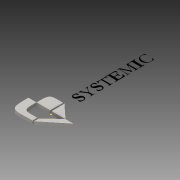
# Autodesk Inventor part: Systemic_Logo
Saved by Autodesk Inventor 2016 (Build 200138000, 138)
## iProperties
Created: 2015-05-10
Part Number: Systemic_Logo
Material: Generic
Document SubType Name: Modeling
Designer: Yann
Density: 1 g/cm^3
Appearance: Aluminum - Polished
Author: Yann
Autodesk Inventor part; units mm, degrees
ref_plane "YZ Plane" through (0, 0, 0) normal (1, 0, 0) x (0, 1, 0)
ref_plane "XZ Plane" through (0, 0, 0) normal (0, 1, 0) x (-1, 0, 0)
ref_plane "XY Plane" through (0, 0, 0) normal (0, 0, 1) x (1, 0, 0)
sketch "Sketch1" plane through (0, 0, 0) normal (0, 1, 0) x (-1, 0, 0)
  line L0 (6.9821, 0) -> (4.4821, 0)
  line L1 (0.2, 4) -> (0.2, 5.5)
  line L2 (-4.4821, 0) -> (-6.9821, 0)
  line L3 (-0.2, 5.5) -> (-0.2, 4)
  line L4 (-10.1992, 0) -> (12.3203, 0) construction
  line L5 (0, -41.6633) -> (0, 16.1649) construction
  line L6 (0.2, 5.5) -> (0.4844, 5.5) construction
  line L7 (0.4844, 5.5) -> (6.9821, 5.5) construction
  line L8 (6.9821, 5.5) -> (6.9821, 6.8061) construction
  line L9 (6.9821, 6.8061) -> (6.9821, 0) construction
  spline S0 degree 4 poles (0.2, 5.5) (0.4844, 5.5) (6.9821, 5.5) (6.9821, 6.8061) (6.9821, 0) knots 1 1 1 1 1 2 2 2 2 2
  line L10 (0.2, 4) -> (1.0687, 4) construction
  line L11 (1.0687, 4) -> (4.4821, 4) construction
  line L12 (4.4821, 4) -> (4.4821, 4.6412) construction
  line L13 (4.4821, 4.6412) -> (4.4821, 0) construction
  spline S1 degree 4 poles (0.2, 4) (1.0687, 4) (4.4821, 4) (4.4821, 4.6412) (4.4821, 0) knots 1 1 1 1 1 2 2 2 2 2
  line L14 (0.2, 4) -> (-0.2, 4) construction
  line L15 (-0.2, 5.5) -> (-6.9821, 0)
  line L16 (4.4821, 0) -> (0.2, 0)
  line L17 (-4.4821, 0) -> (-0.2, 0)
  line L18 (-0.2, 0) -> (-0.2, -4)
  line L19 (-0.2, -4) -> (-4.4821, 0)
  line L20 (0.2, -4) -> (1.0687, -4) construction
  line L21 (1.0687, -4) -> (4.4821, -4) construction
  line L22 (4.4821, -4) -> (4.4821, -4.6412) construction
  line L23 (4.4821, -4.6412) -> (4.4821, 0) construction
  spline S2 degree 4 poles (0.2, -4) (1.0687, -4) (4.4821, -4) (4.4821, -4.6412) (4.4821, 0) knots 1 1 1 1 1 2 2 2 2 2
  line L24 (0.2, 0) -> (0.2, -4)
  line L25 (-0.2, -4) -> (0.2, -4) construction
  line L26 (-4.4821, 0) -> (-0.2, 4)
  point P0 (0, 0)
  dimension "d0" = 0.2
  dimension "d1" = 4
  dimension "d3" = 2.5
  dimension "d6" = 1.5
  constraints: 26 end point, 5 perpendicular, 5 symmetric about line, 4 horizontal, 4 point on line, 4 vertical, 2 collinear, 2 equal length, 1 parallel, 11 other
  measures "d0" distance between parallel lines of L5 L1
  measures "d1" vertical distance of L1.start point (0, 0)
  measures "d3" distance of L2.start L2.end
  measures "d6" distance of L3.start L3.end
extrude "Extrusion1" add sketch "Sketch1" along normal blind 1
sketch "Sketch2" plane through (0, 0, 0) normal (0, 1, 0) x (-1, 0, 0)
  line L0 (0, -40.0826) -> (0, 6.6804) construction
  line L1 (-5.6893, 0) -> (7.9729, 0) construction
  spline S0 degree 4 poles (5.7309, -9.156) (6.4153, -8.9173) (4.9983, -7.4481) (5.0462, -8.6728) (4.0888, -9.5797) (3.7167, -8.7652) (3.7309, -8.156) knots 0 0 0 0 0 0.475399 0.676528 1 1 1 1 1
  line L2 (3.7203, -8.6135) -> (3.7416, -7.6985) construction
  arc A0 (3.7712, -7.7964) -> (3.7544, -8.5171) centre (5.7845, -8.2039) ccw construction
  point P0 (0, 0)
  point P1 (2.7309, -8.156)
  point P2 (2.7309, -9.156)
  point P3 (3.7309, -9.156)
  point P4 (4.7309, -8.156)
  point P5 (4.7309, -9.156)
  point P6 (5.7309, -8.156)
  point P7 (2.7309, -10.156)
  point P8 (3.7309, -10.156)
  point P9 (4.7309, -10.156)
  point P10 (5.7309, -10.156)
  point P11 (2.7309, -11.156)
  point P12 (3.7309, -11.156)
  point P13 (4.7309, -11.156)
  point P14 (5.7309, -11.156)
  point P15 (2.7309, -12.156)
  point P16 (3.7309, -12.156)
  point P17 (4.7309, -12.156)
  point P18 (5.7309, -12.156)
  point P19 (2.7309, -13.156)
  point P20 (3.7309, -13.156)
  point P21 (4.7309, -13.156)
  point P22 (5.7309, -13.156)
  point P23 (2.7309, -14.156)
  point P24 (3.7309, -14.156)
  point P25 (4.7309, -14.156)
  point P26 (5.7309, -14.156)
  point P27 (2.7309, -15.156)
  point P28 (3.7309, -15.156)
  point P29 (4.7309, -15.156)
  point P30 (5.7309, -15.156)
  point P31 (2.7309, -16.156)
  point P32 (3.7309, -16.156)
  point P33 (4.7309, -16.156)
  point P34 (5.7309, -16.156)
  point P35 (2.7309, -17.156)
  point P36 (3.7309, -17.156)
  point P37 (4.7309, -17.156)
  point P38 (5.7309, -17.156)
  point P39 (2.7309, -18.156)
  point P40 (3.7309, -18.156)
  point P41 (4.7309, -18.156)
  point P42 (5.7309, -18.156)
  point P43 (2.7309, -19.156)
  point P44 (3.7309, -19.156)
  point P45 (4.7309, -19.156)
  point P46 (5.7309, -19.156)
  point P47 (2.7309, -20.156)
  point P48 (3.7309, -20.156)
  point P49 (4.7309, -20.156)
  point P50 (5.7309, -20.156)
  point P51 (2.7309, -21.156)
  point P52 (3.7309, -21.156)
  point P53 (4.7309, -21.156)
  point P54 (5.7309, -21.156)
  point P55 (2.7309, -22.156)
  point P56 (3.7309, -22.156)
  point P57 (4.7309, -22.156)
  point P58 (5.7309, -22.156)
  point P59 (2.7309, -23.156)
  point P60 (3.7309, -23.156)
  point P61 (4.7309, -23.156)
  point P62 (5.7309, -23.156)
  point P63 (2.7309, -24.156)
  point P64 (3.7309, -24.156)
  point P65 (4.7309, -24.156)
  point P66 (5.7309, -24.156)
  point P67 (2.7309, -25.156)
  point P68 (3.7309, -25.156)
  point P69 (4.7309, -25.156)
  point P70 (5.7309, -25.156)
  point P71 (2.7309, -26.156)
  point P72 (3.7309, -26.156)
  point P73 (4.7309, -26.156)
  point P74 (5.7309, -26.156)
  point P75 (2.7309, -27.156)
  point P76 (3.7309, -27.156)
  point P77 (4.7309, -27.156)
  point P78 (5.7309, -27.156)
  point P79 (2.7309, -28.156)
  point P80 (3.7309, -28.156)
  point P81 (4.7309, -28.156)
  point P82 (5.7309, -28.156)
  point P83 (5.7309, -8.4151)
  point P84 (5.1242, -8.156)
  point P85 (4.7309, -8.7206)
  point P86 (4.2129, -9.1858)
  point P87 (5.6724, -8.9882)
  point P88 (3.5533, -8.1518)
  dimension "d9" = 1
  dimension "d12" = 1
  constraints: 2 end point, 2 midpoint, 1 centre point, 1 horizontal, 1 point on circle, 1 vertical, 94 other
  measures "d9" distance of point (2.731, -8.156) point (3.731, -8.156)
  measures "d12" distance of point (2.731, -8.156) point (2.731, -9.156)
sketch "Sketch3" plane through (0, 0, 0) normal (0, 1, 0) x (-1, 0, 0)
  line L0 (1.8486, -7.6205) -> (1.8486, -33.4021) construction
  line L1 (1.8486, -33.4021) -> (-3.7375, -33.4021) construction
  line L2 (-3.7375, -33.4021) -> (-3.7375, -7.6205) construction
  line L3 (-3.7375, -7.6205) -> (1.8486, -7.6205) construction
  point P0 (0, 0)
  constraints: 2 other
body "Solid1"
